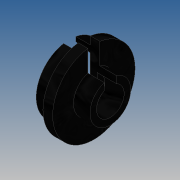
# Autodesk Inventor part: Rondelle
Saved by Autodesk Inventor 2021.3 (Build 253353000, 353)
## iProperties
Created: 2023-04-12
Part Number: Rondelle
Material: ABS Plastic
Document SubType Name: Modeling
Designer: cedric.clivaz
Density: 1.06 g/cm^3
Appearance: Black
Author: cedric.clivaz
Autodesk Inventor part; units mm, degrees
ref_plane "YZ Plane" through (0, 0, 0) normal (1, 0, 0) x (0, 1, 0)
ref_plane "XZ Plane" through (0, 0, 0) normal (0, 1, 0) x (-1, 0, 0)
ref_plane "XY Plane" through (0, 0, 0) normal (0, 0, 1) x (1, 0, 0)
sketch "Sketch2" plane through (0, 0, 0) normal (0, 0, 1) x (1, 0, 0)
  line L0 (0, -1.7) -> (0, 10.2) construction
  line L1 (-1.68, 0) -> (10.08, 0) construction
  line L2 (8.4, 2.85) -> (8.4, 4.2)
  line L3 (8.4, 4.2) -> (5, 4.2)
  line L4 (5, 4.2) -> (5, 8.5)
  line L5 (5, 8.5) -> (3, 8.5)
  line L6 (3, 8.5) -> (3, 6.9)
  line L7 (3, 6.9) -> (0, 6.9)
  line L8 (0, 6.9) -> (0, 6)
  line L9 (0, 6) -> (3, 5.5)
  line L10 (3, 5.5) -> (3, 2.85)
  line L11 (8.4, 2.85) -> (4.4, 2.85)
  line L12 (4.4, 2.85) -> (4.4, 1.6)
  line L13 (4.4, 1.6) -> (3, 1.6)
  line L14 (3, 1.6) -> (3, 2.85)
  point P0 (0, 0)
  dimension "d0" = 17
  dimension "d1" = 8.4
  dimension "d2" = 8.4
  dimension "d3" = 3.4
  dimension "d5" = 13.8
  dimension "d6" = 11
  dimension "d7" = 12
  dimension "d8" = 3
  dimension "d9" = 3
  dimension "d11" = 5.7
  dimension "d12" = 4
  dimension "d13" = 3.2
  constraints: 26 end point, 9 perpendicular, 1 collinear, 1 horizontal, 1 parallel, 1 vertical
  measures "d0" diameter of L5 L1
  measures "d1" diameter of L3 L1
  measures "d2" distance between parallel lines of L8 L2
  measures "d3" distance between parallel lines of L2 L4
  measures "d5" diameter of L7 L1
  measures "d6" diameter of L9.end L1
  measures "d7" diameter of L8.end L1
  measures "d8" distance between parallel lines of L6 L8
  measures "d9" distance between parallel lines of L10 L8
  measures "d11" diameter of L11 L1
  measures "d12" distance between parallel lines of L2 L12
  measures "d13" diameter of L13 L1
revolve "Revolution1" add sketch "Sketch2" angle 360 about axis through (-10, 0, 0) along (1, 0, 0)
sketch "Sketch3" plane through (0, 0, 0) normal (0, 0, 1) x (1, 0, 0)
  line L0 (-1.68, 0) -> (10.08, 0) construction
  line L1 (0, -6.9) -> (0, 6.9) construction
  line L2 (8.4, -4.2) -> (8.4, 4.2) construction
  line L3 (0, 1.25) -> (8.4, 1.25)
  line L4 (8.4, 1.25) -> (8.4, -1.25)
  line L5 (8.4, -1.25) -> (0, -1.25)
  line L6 (0, -1.25) -> (0, 1.25)
  point P0 (0, 0)
  dimension "d14" = 2.5
  constraints: 8 end point, 2 parallel, 2 point on line, 1 horizontal, 1 perpendicular, 1 other
  measures "d14" distance between parallel lines of L5 L3
extrude "Extrusion1" cut sketch "Sketch3" along normal through all
body "Solid1"
